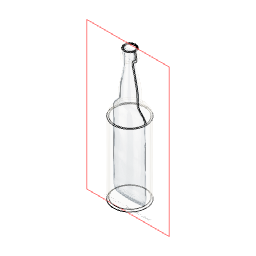
glass soda bottle v2 (Autodesk Fusion 360 design; units mm, degrees)
Autodesk Fusion 360 part; units mm, degrees
sketch "Sketch1" plane through (0, 0, 0) normal (0, 1, 0) x (1, 0, 0) in component "bottle"
  line L0 (0, 0) -> (0, -240)
  line L1 (0, 0) -> (30, 0)
  line L2 (30, 0) -> (30, -1)
  line L3 (30, -1) -> (30, -131)
  spline S0 degree 5 poles (30, -131) (30, -131.5768) (29.9387, -132.7187) (29.6631, -134.3959) (28.9442, -136.5521) (27.5606, -139.0676) (25.8335, -141.3536) (23.9245, -143.379) (21.9966, -145.1496) (20.1923, -146.7353) (18.6212, -148.267) (17.3585, -149.8999) (16.4393, -151.7846) (15.856, -154.0366) (15.5524, -156.7038) (15.4396, -159.7758) (15.413, -163.1955) (15.3681, -166.8694) (15.2177, -170.6786) (14.9065, -174.4896) (14.4325, -178.1642) (13.8458, -181.5729) (13.2215, -184.6137) (12.64, -187.2278) (12.1617, -189.4194) (11.8091, -191.2693) (11.5356, -192.9627) (11.2319, -194.7693) (10.7796, -196.9545) (10.0952, -199.7075) (9.1761, -203.0635) (8.1499, -206.8235) (7.2221, -210.6413) (6.6198, -214.1223) (6.5378, -216.9133) (7.0796, -218.8041) (8.2112, -219.8066) (9.6807, -220.2901) (11.1163, -220.822) (12.1678, -221.9335) (12.6646, -223.8606) (12.6348, -226.513) (12.224, -229.6106) (11.6426, -232.7718) (11.1065, -235.6139) (10.7688, -237.8671) (10.7142, -239.0986) (10.8057, -239.6816) (10.9254, -239.9191) (11, -240) knots 0 0 0 0 0 0 0.022222 0.044444 0.066667 0.088889 0.111111 0.133333 0.155556 0.177778 0.2 0.222222 0.244444 0.266667 0.288889 0.311111 0.333333 0.355556 0.377778 0.4 0.422222 0.444444 0.466667 0.488889 0.511111 0.533333 0.555556 0.577778 0.6 0.622222 0.644444 0.666667 0.688889 0.711111 0.733333 0.755556 0.777778 0.8 0.822222 0.844444 0.866667 0.888889 0.911111 0.933333 0.955556 0.977778 1 1 1 1 1 1
  line L4 (0, -240) -> (11, -240)
  point P0 (22.9095, -144.2909)
  point P1 (16.4738, -152.0138)
  point P2 (15.0257, -172.769)
  point P3 (11.9688, -190.4673)
  point P4 (10, -200)
  point P5 (7.4638, -218.9454)
  point P6 (11.4861, -221.3588)
  point P7 (11.3822, -234.1778)
  dimension "d1" = 240
  dimension "d2" = 30
  dimension "d3" = 1
  dimension "d4" = 130
  dimension "d5" = 11
  constraint coincident L0.start L1.start
  constraint vertical L0
  constraint perpendicular L0 L1
  constraint vertical L2
  constraint perpendicular L1 L3
  constraint perpendicular L0 L4
  measures "d1" distance of L0.start L0.end
  measures "d2" distance of L0.start L1.end
  measures "d3" distance of L1.end L2.end
  measures "d4" distance of L2.end L3.end
  measures "d5" distance of L0.end S0.end
revolve "Revolve1" add sketch "Sketch1" angle 360 about axis through (0, 0, 0) along (0, 0, 1) in component "bottle"
shell "Shell1" thickness 2.5 removed faces 1 at (1.9764, -3.8951, 240) in component "bottle"
fillet "Fillet1" radius 1 1 edges at (-10.2556, -3.9778, 240) in component "bottle"
fillet "Fillet2" radius 1 1 edges at (-8.3552, 0.0033, 240) in component "bottle"
component "bottle" placed x (1, 0, 0) y (0, 1, 0) z (0, 0, 1) at (0, 0, 0)
